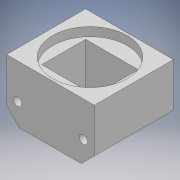
# Autodesk Inventor part: drive R
Saved by Autodesk Inventor 2017 (Build 210142000, 142)
## iProperties
Created: 2018-08-02
Part Number: drive R
Material: Generic
Document SubType Name: Modeling
Designer: jakub.tomczynski
Density: 1 g/cm^3
Appearance: Default
Author: jakub.tomczynski
Autodesk Inventor part; units mm, degrees
ref_plane "YZ Plane" through (0, 0, 0) normal (1, 0, 0) x (0, 1, 0)
ref_plane "XZ Plane" through (0, 0, 0) normal (0, 1, 0) x (-1, 0, 0)
ref_plane "XY Plane" through (0, 0, 0) normal (0, 0, 1) x (1, 0, 0)
sketch "Sketch1" plane through (0, 0, 0) normal (0, 0, 1) x (1, 0, 0)
  line L0 (0, 0) -> (20, 0)
  line L1 (20, 0) -> (20, 18)
  line L2 (20, 18) -> (0, 18)
  line L3 (0, 18) -> (0, 0)
  dimension "d0" = 20
  dimension "d1" = 18
  constraints: 8 end point, 2 parallel, 1 horizontal, 1 perpendicular
  measures "d0" distance of L2.end L1.end
  measures "d1" distance of L1.end L0.end
extrude "body" add sketch "Sketch1" along normal blind 13
sketch "Sketch2" plane through (0, 18, 0) normal (0, 1, 0) x (1, 0, 0)
  line L0 (20, 0) -> (0, 0) projected
  point P0 (2.5, -5)
  point P1 (17.5, -5)
  dimension "d4" = 2.5
  dimension "d5" = 2.5
  dimension "d6" = 5
  dimension "d7" = 5
  measures "d4" horizontal distance of point (2.5, -5) L0.end
  measures "d5" horizontal distance of L0.start point (17.5, -5)
  measures "d6" vertical distance of L0.start point (17.5, -5)
  measures "d7" vertical distance of L0.end point (2.5, -5)
hole "top mount" at (2.5, 18, 5) at (17.5, 18, 5) direction (0, -1, 0) diameter 1.9 depth 4
sketch "Sketch3" plane through (0, 0, 0) normal (0, -1, 0) x (1, 0, 0)
  line L0 (0, 0) -> (20, 0) projected
  point P0 (17.5, 5)
  point P1 (2.5, 5)
  dimension "d15" = 5
  dimension "d16" = 5
  dimension "d17" = 2.5
  dimension "d18" = 2.5
  measures "d15" vertical distance of L0.end point (17.5, 5)
  measures "d16" vertical distance of L0.start point (2.5, 5)
  measures "d17" horizontal distance of L0.start point (2.5, 5)
  measures "d18" horizontal distance of L0.end point (17.5, 5)
hole "bottom mount" at (17.5, 0, 5) at (2.5, 0, 5) direction (0, 1, 0) diameter 1.9 depth 4
sketch "Sketch4" plane through (0, 0, 13) normal (0, 0, 1) x (1, 0, 0)
  point P0 (0, 0)
  point P1 (0, 18)
  point P2 (10, 9)
  dimension "d26" = 10
  dimension "d27" = 9
  measures "d26" horizontal distance of point (0, 18) point (10, 9)
  measures "d27" vertical distance of point (10, 9) point (0, 18)
hole "spool" at (10, 9, 13) direction (0, 0, -1) diameter 17 depth 2
sketch "Sketch5" plane through (0, 0, 13) normal (0, 0, 1) x (1, 0, 0)
  line L0 (4, 4) -> (16, 4)
  line L1 (16, 4) -> (16, 14)
  line L2 (16, 14) -> (4, 14)
  line L3 (4, 14) -> (4, 4)
  line L4 (4, 4) -> (16, 14) construction
  line L5 (16, 4) -> (4, 14) construction
  point P0 (0, 0)
  point P1 (10, 9)
  dimension "d35" = 12
  dimension "d36" = 10
  constraints: 12 end point, 2 midpoint, 2 parallel, 1 horizontal, 1 perpendicular
  measures "d35" distance of L2.end L1.end
  measures "d36" distance of L1.end L0.end
extrude "gearbox pocket" cut sketch "Sketch5" against normal blind 12
sketch "Sketch6" plane through (0, 0, 1) normal (0, 0, 1) x (1, 0, 0)
  line L0 (13.3166, 4) -> (6.6834, 4)
  line L1 (6.6834, 4) -> (6.6834, 14)
  line L2 (6.6834, 14) -> (13.3166, 14)
  line L3 (13.3166, 14) -> (13.3166, 4)
  line L4 (13.3166, 4) -> (6.6834, 14) construction
  line L5 (6.6834, 4) -> (13.3166, 14) construction
  arc A0 (13.3166, 4) -> (13.3166, 14) centre (10, 9) ccw
  arc A1 (6.6834, 4) -> (13.3166, 4) centre (10, 9) ccw construction
  arc A2 (13.3166, 14) -> (6.6834, 14) centre (10, 9) ccw construction
  arc A3 (6.6834, 14) -> (6.6834, 4) centre (10, 9) ccw
  dimension "d46" = 12
  dimension "d47" = 10
  constraints: 12 end point, 8 point on circle, 4 centre point, 2 parallel, 1 coincident, 1 horizontal, 1 perpendicular
  measures "d46" diameter of A0
  measures "d47" distance between parallel lines of L2 L0
extrude "Extrusion3" cut sketch "Sketch6" against normal through all
chamfer "Chamfer1" distance 3 angle 45 2 edges at (0, 9, 0) (20, 9, 0)
body "Solid1"
